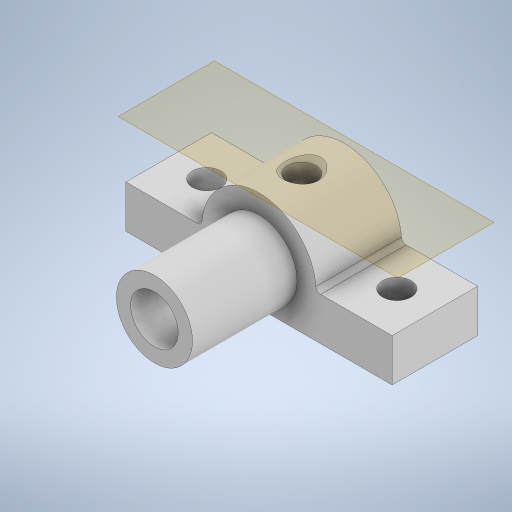
# Autodesk Inventor part: Hudson 1-71
Saved by Autodesk Inventor 2024.2 (Build 282272000, 272)
## iProperties
Created: 2024-10-10
Part Number: Hudson 1-71
Material: Generic
Document SubType Name: Modeling
Designer: Precisión-12
Density: 1 g/cm^3
Appearance: Default
Author: Precisión-12
Autodesk Inventor part; units mm, degrees
ref_plane "YZ Plane" through (0, 0, 0) normal (1, 0, 0) x (0, 1, 0)
ref_plane "XZ Plane" through (0, 0, 0) normal (0, 1, 0) x (-1, 0, 0)
ref_plane "XY Plane" through (0, 0, 0) normal (0, 0, 1) x (1, 0, 0)
sketch "Sketch1" plane through (0, 0, 0) normal (0, 0, 1) x (1, 0, 0)
  line L0 (14, 0) -> (-14, 0)
  line L1 (-14, 0) -> (-14, -4.5)
  line L2 (-14, -4.5) -> (14, -4.5)
  line L3 (14, -4.5) -> (14, 0)
  line L4 (0, 29.3592) -> (0, -29.3592) construction
  arc A0 (5.9822, 0.4615) -> (-5.9822, 0.4615) centre (0, 0) ccw
  circle A1 centre (0, 0) radius 2.5
  circle A2 centre (0, 0) radius 4
  arc A3 (5.9822, 0.4615) -> (6.4807, 0) centre (6.4807, 0.5) ccw
  arc A4 (-6.4807, 0) -> (-5.9822, 0.4615) centre (-6.4807, 0.5) ccw
  dimension "d0" = 14
  dimension "d1" = 4.5
  dimension "d2" = 12
  dimension "d3" = 8
  dimension "d4" = 5
  dimension "d5" = 1
  dimension "d6" = 1
  constraints: 10 end point, 6 point on circle, 5 centre point, 4 coincident, 4 tangent, 2 midpoint, 2 parallel, 2 point on line, 1 horizontal, 1 perpendicular, 1 vertical
  measures "d0" distance between parallel lines of L4 L3
  measures "d1" distance of L0.end L1.end
  measures "d2" diameter of A0
  measures "d3" diameter of A2
  measures "d4" diameter of A1
  measures "d5" diameter of A3
  measures "d6" diameter of A4
extrude "Extrusion1" add sketch "Sketch1" along normal blind 9 contours L3 L2 L1 L0 A2 | L0 A2 A4 A0 A3
extrude "Extrusion2" add sketch "Sketch1" along normal blind 20 contours A2 L0 A1 | L0 A1 A2
ref_plane "Plano de trabajo2" through (-14, 6, 0) normal (0, 1, 0) x (1, 0, 0)
sketch "Boceto3" plane through (-14, 6, 0) normal (0, 1, 0) x (1, 0, 0)
  line L0 (14, 0) -> (14, -9) construction
  line L1 (8.0178, -9) -> (19.9822, -9) projected
  line L2 (0, 0) -> (0, -9) projected
  line L3 (0, -4.5) -> (28, -4.5) construction
  line L4 (28, 0) -> (28, -9) projected
  circle A0 centre (4, -4.5) radius 1.5
  circle A1 centre (14, -4.5) radius 1.5
  circle A2 centre (24, -4.5) radius 1.5
  line L5 (7.5193, 0) -> (0, 0) projected
  line L6 (0, 0) -> (0, -9) projected
  line L7 (7.5193, -9) -> (0, -9) projected
  line L8 (7.5193, 0) -> (7.5193, -9) projected
  line L9 (19.9822, 0) -> (8.0178, 0) projected
  line L10 (8.0178, 0) -> (8.0178, -9) projected
  line L11 (19.9822, -9) -> (8.0178, -9) projected
  line L12 (19.9822, 0) -> (19.9822, -9) projected
  line L13 (28, 0) -> (20.4807, 0) projected
  line L14 (20.4807, 0) -> (20.4807, -9) projected
  line L15 (28, -9) -> (20.4807, -9) projected
  line L16 (28, 0) -> (28, -9) projected
  dimension "d25" = 3
  dimension "d26" = 3
  dimension "d27" = 3
  dimension "d28" = 10
  dimension "d29" = 10
  constraints: 4 end point, 4 midpoint, 3 centre point, 2 point on line, 1 coincident
  measures "d25" diameter of A0
  measures "d26" diameter of A1
  measures "d27" diameter of A2
  measures "d28" distance from line of L0 A0.centre
  measures "d29" distance from line of L0 A2.centre
hole "Agujero2" at (0, 6, 4.5) direction (0, -1, 0) diameter 3 depth 5 countersink diameter 4 countersink angle 90
hole "Agujero3" at (-10, 6, 4.5) at (10, 6, 4.5) direction (0, -1, 0) diameter 3 end through all
body "Solid1"
